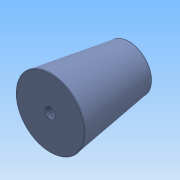
# Autodesk Inventor part: ножки
Saved by Autodesk Inventor 2017 (Build 210142000, 142)
## iProperties
Part Number: ножки
Material: Типовые
Document SubType Name: Modeling
Designer: Max
Mass: 9.96625 g
Surface Area: 33.7955 cm^2
Volume: 9.96625 cm^3
Density: 1 g/cm^3
Appearance: Резина — синяя
Author: Max
Autodesk Inventor part; units mm, degrees
ref_plane "YZ Plane" through (0, 0, 0) normal (1, 0, 0) x (0, 1, 0)
ref_plane "XZ Plane" through (0, 0, 0) normal (0, 1, 0) x (-1, 0, 0)
ref_plane "XY Plane" through (0, 0, 0) normal (0, 0, 1) x (1, 0, 0)
sketch "Эскиз1" plane through (0, 0, 0) normal (0, 0, 1) x (1, 0, 0)
  line L0 (0, 0) -> (0, 30)
  line L1 (3.9, 30) -> (8.5, 30)
  line L2 (8.5, 30) -> (13, 0)
  line L3 (0, 0) -> (13, 0)
  line L4 (3.9, 30) -> (3.9, 10)
  line L5 (3.9, 10) -> (2, 10)
  line L6 (2, 10) -> (2, 0)
  dimension "d0" = 30
  dimension "d1" = 4
  dimension "d2" = 7.8
  dimension "d3" = 17
  dimension "d4" = 26
  dimension "d8" = 10
  constraints: 14 end point, 3 perpendicular, 2 point on line, 2 vertical, 1 parallel
  measures "d0" distance of L0.start L0.end
  measures "d1" diameter of L6 L0
  measures "d2" diameter of L4 L0
  measures "d3" diameter of L1.end L0
  measures "d4" diameter of L2.end L0
  measures "d8" distance between parallel lines of L3 L5
revolve "Вращение1" add sketch "Эскиз1" angle 360 about axis through (0, 0, 0) along (0, 1, 0)
fillet "Сопряжение1" radius 0.2 1 edges at (-13, 0, 0)
fillet "Сопряжение2" radius 0.5 1 edges at (-8.5, 30, 0)
